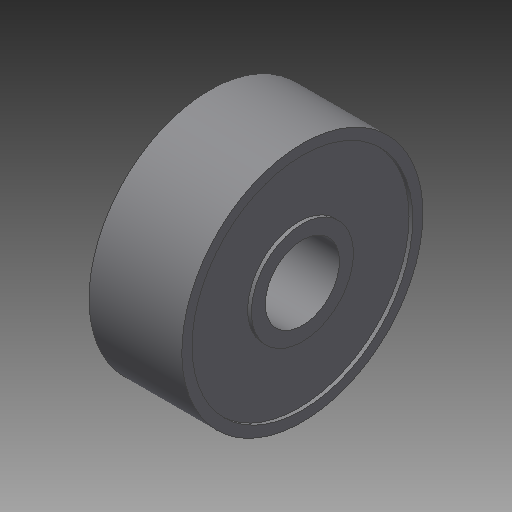
# Autodesk Inventor part: riku_mae_bis17_624-ZZ-MAE
Saved by Autodesk Inventor 2019.1 (Build 231200000, 200)
## iProperties
Category: PARTsolutions
Company: MAEDLER
Created: 2018-08-16
Part Number: riku_mae_bis17_624-ZZ-MAE
Material: Allgemein
Catalog Web Link: www.cadenas.de
Description: riku_mae_bis17-Single Row Deep Groove Ball Bearings MÄDLER
Vendor: MAEDLER
Document SubType Name: Modeling
Designer: psadmin
Manufacturer: MAEDLER
Mass: 3 g
Surface Area: 5.29233 cm^2
Volume: 0.565845 cm^3
Density: 1 g/cm^3
Appearance: PSOLRGB-175-175-175
PSOL_IDENT_0: {$CADENAS_DATA\23d-libs\maedler\antriebselemente\kugellager\maedler_klager\riku_mae_bis17.prj},198 {
PSOL_IDENT_1: VTYP=3D},{NB=riku_mae_bis17_624-ZZ-MAE},{LINA=riku_mae_bis17_624-ZZ-MAE},{NN=riku_mae_bis17},{DATE=3
PSOL_IDENT_2: 0.05.2018 06:10:28},{GEOMDATE=30.05.2018 06:10:28},{VERSION=},{LINEID=30},{WBVAR=},{WBNUMERIC=}  {NB=
PSOL_IDENT_3: riku_mae_bis17_624-ZZ-MAE},{LINA=riku_mae_bis17_624-ZZ-MAE},{KT=DUMMY},{ARTNR=624-ZZ-MAE},{LG1=Lager
PSOL_IDENT_4: luft CN},{PDF=PDF-Katalogseite},{D1=4.000},{D2=13.000},{B=5.000},{AUSF=beidseitig Deckscheiben},{DYN=
PSOL_IDENT_5: 1,30},{STAT=0,49},{GRENZD=40.000},{GEW=3.00},{D3=5.500},{D4=11.900},{RS=0.200}
NN: riku_mae_bis17
NT: Rillenkugellager MÄDLER®, einreihig, Innendurchmesser 3 bis 17 mm, Lagerluft CN und C3
NB: riku_mae_bis17_624-ZZ-MAE
NBSYN: riku_mae_bis17_$ARTNR.
LINA: riku_mae_bis17_624-ZZ-MAE
ARTNR: 624-ZZ-MAE
LG1: Lagerluft CN
PDF: PDF-Katalogseite
D1: 4
D2: 13
B: 5
AUSF: beidseitig Deckscheiben
DYN: 1,30
STAT: 0,49
GRENZD: 40.000
GEW: 3
SUPPLIER: MAEDLER
ARTICLENO: riku_mae_bis17_624-ZZ-MAE
BOMINFO: riku_mae_bis17_624-ZZ-MAE
CREATOR: CADENAS GmbH
Title: riku_mae_bis17_624-ZZ-MAE
Author: Cadenas PARTsolutions
Comments: Single Row Deep Groove Ball Bearings MÄDLER
Autodesk Inventor part; units mm, degrees
ref_plane "YZ Plane" through (0, 0, 0) normal (1, 0, 0) x (0, 1, 0)
ref_plane "XZ Plane" through (0, 0, 0) normal (0, 1, 0) x (-1, 0, 0)
ref_plane "XY Plane" through (0, 0, 0) normal (0, 0, 1) x (1, 0, 0)
sketch "Sketch_1" plane through (0, 0, 0) normal (0, 0, 1) x (1, 0, 0)
  line L0 (50, 0) -> (-50, 0)
  line L1 (-2.5, 5.95) -> (-2.3, 5.95)
  line L2 (-2.3, 5.95) -> (-2.3, 2.75)
  line L3 (-2.3, 2.75) -> (-2.5, 2.75)
  line L4 (-2.5, 2.75) -> (-2.5, 2)
  line L5 (-2.5, 2) -> (2.5, 2)
  line L6 (2.5, 2) -> (2.5, 2.75)
  line L7 (2.5, 2.75) -> (2.3, 2.75)
  line L8 (2.3, 2.75) -> (2.3, 5.95)
  line L9 (2.3, 5.95) -> (2.5, 5.95)
  line L10 (2.5, 5.95) -> (2.5, 6.5)
  line L11 (2.5, 6.5) -> (-2.5, 6.5)
  line L12 (-2.5, 6.5) -> (-2.5, 5.95)
  constraints: 26 end point
revolve "Revolution1" add sketch "Sketch_1" angle 360 about axis through (50, 0, 0) along (1, 0, 0)
body "Solid1"
